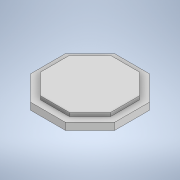
# Autodesk Inventor part: SatelliteBottomFace
Saved by Autodesk Inventor 2020 (Build 240168000, 168)
## iProperties
Created: 2020-02-24
Part Number: SatelliteBottomFace
Material: Generic
Document SubType Name: Modeling
Designer: WANG
Density: 1 g/cm^3
Appearance: Default
Author: WANG
Autodesk Inventor part; units mm, degrees
ref_plane "YZ Plane" through (0, 0, 0) normal (1, 0, 0) x (0, 1, 0)
ref_plane "XZ Plane" through (0, 0, 0) normal (0, 1, 0) x (-1, 0, 0)
ref_plane "XY Plane" through (0, 0, 0) normal (0, 0, 1) x (1, 0, 0)
sketch "Sketch1" plane through (0, 0, 0) normal (0, 1, 0) x (-1, 0, 0)
  line L0 (0, 0) -> (152.4, 0) construction
  line L1 (152.4, 0) -> (152.4, -152.4) construction
  line L2 (152.4, -152.4) -> (0, -152.4) construction
  line L3 (0, -152.4) -> (0, 0) construction
  line L4 (44.6369, -152.4) -> (0, -107.7631)
  line L5 (0, -107.7631) -> (0, -44.6369)
  line L6 (0, -44.6369) -> (44.6369, 0)
  line L7 (44.6369, 0) -> (107.7631, 0)
  line L8 (107.7631, 0) -> (152.4, -44.6369)
  line L9 (152.4, -44.6369) -> (152.4, -107.7631)
  line L10 (152.4, -107.7631) -> (107.7631, -152.4)
  line L11 (107.7631, -152.4) -> (44.6369, -152.4)
  line L12 (102.5026, -12.7) -> (139.7, -49.8974)
  line L13 (139.7, -49.8974) -> (139.7, -102.5026)
  line L14 (139.7, -102.5026) -> (102.5026, -139.7)
  line L15 (102.5026, -139.7) -> (49.8974, -139.7)
  line L16 (49.8974, -139.7) -> (12.7, -102.5026)
  line L17 (12.7, -102.5026) -> (12.7, -49.8974)
  line L18 (12.7, -49.8974) -> (49.8974, -12.7)
  line L19 (49.8974, -12.7) -> (102.5026, -12.7)
  point P0 (76.2, -76.2)
  point P1 (76.2, -76.2)
  point P2 (76.2, -76.2)
  dimension "d0" = 152.4
  dimension "d1" = 152.4
  dimension "d2" = 12.7
  dimension "d3" = 63.1262
  dimension "d4" = 52.6051
  constraints: 40 end point, 3 collinear, 2 coincident, 2 horizontal, 2 parallel, 1 perpendicular, 1 point on line, 34 other
  measures "d0" distance of L1.end L2.end
  measures "d1" distance of L0.end L1.end
  measures "d2" distance between parallel lines of L13 L9
  measures "d3" distance of L9.end L10.end
  measures "d4" distance of L13.end L14.end
sketch "Sketch2" plane through (0, 0, 0) normal (0, 1, 0) x (-1, 0, 0)
  line L0 (0, 0) -> (152.4, 0) construction
  line L1 (152.4, 0) -> (152.4, -152.4) construction
  line L2 (152.4, -152.4) -> (0, -152.4) construction
  line L3 (0, -152.4) -> (0, 0) construction
  line L4 (44.6369, -152.4) -> (0, -107.7631)
  line L5 (0, -107.7631) -> (0, -44.6369)
  line L6 (0, -44.6369) -> (44.6369, 0)
  line L7 (44.6369, 0) -> (107.7631, 0)
  line L8 (107.7631, 0) -> (152.4, -44.6369)
  line L9 (152.4, -44.6369) -> (152.4, -107.7631)
  line L10 (152.4, -107.7631) -> (107.7631, -152.4)
  line L11 (107.7631, -152.4) -> (44.6369, -152.4)
  line L12 (102.5026, -12.7) -> (139.7, -49.8974)
  line L13 (139.7, -49.8974) -> (139.7, -102.5026)
  line L14 (139.7, -102.5026) -> (102.5026, -139.7)
  line L15 (102.5026, -139.7) -> (49.8974, -139.7)
  line L16 (49.8974, -139.7) -> (12.7, -102.5026)
  line L17 (12.7, -102.5026) -> (12.7, -49.8974)
  line L18 (12.7, -49.8974) -> (49.8974, -12.7)
  line L19 (49.8974, -12.7) -> (102.5026, -12.7)
  point P0 (76.2, -76.2)
  point P1 (76.2, -76.2)
  point P2 (76.2, -76.2)
  dimension "d5" = 152.4
  dimension "d6" = 152.4
  dimension "d7" = 12.7
  dimension "d8" = 63.1262
  dimension "d9" = 52.6051
  constraints: 40 end point, 3 collinear, 2 coincident, 2 horizontal, 2 parallel, 1 perpendicular, 1 point on line, 34 other
  measures "d5" distance of L1.end L2.end
  measures "d6" distance of L0.end L1.end
  measures "d7" distance between parallel lines of L13 L9
  measures "d8" distance of L9.end L10.end
  measures "d9" distance of L13.end L14.end
extrude "Extrusion1" add sketch "Sketch1" along normal blind 12.7 contours L4 L5 L6 L7 L8 L9 L10 L11 | L12 L13 L14 L15 L16 L17 L18 L19
extrude "Extrusion2" add sketch "Sketch2" along normal blind 19.05 contours L12 L13 L14 L15 L16 L17 L18 L19
body "Solid1"
